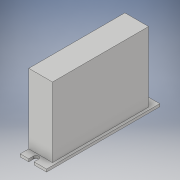
# Autodesk Inventor part: DM332T_Stepper
Saved by Autodesk Inventor 2019.4 (Build 234330000, 330)
## iProperties
Created: 2021-02-07
Part Number: DM332T_Stepper
Material: Generic
Document SubType Name: Modeling
Designer: Jorian Brusind
Density: 1 g/cm^3
Appearance: Default
Author: Jorian Brusind
Autodesk Inventor part; units mm, degrees
ref_plane "YZ Plane" through (0, 0, 0) normal (1, 0, 0) x (0, 1, 0)
ref_plane "XZ Plane" through (0, 0, 0) normal (0, 1, 0) x (-1, 0, 0)
ref_plane "XY Plane" through (0, 0, 0) normal (0, 0, 1) x (1, 0, 0)
sketch "Sketch1" plane through (0, 0, 0) normal (0, 1, 0) x (-1, 0, 0)
  line L0 (0, 0) -> (20, 0)
  line L1 (20, 0) -> (20, -86)
  line L2 (20, -86) -> (0, -86)
  line L3 (0, -86) -> (0, 0)
  dimension "d0" = 20
  dimension "d1" = 86
  constraints: 8 end point, 2 parallel, 1 horizontal, 1 perpendicular
  measures "d0" distance of L1.end L2.end
  measures "d1" distance of L0.end L1.end
extrude "Extrusion1" add sketch "Sketch1" along normal blind 2
sketch "Sketch2" plane through (0, 2, 0) normal (0, 1, 0) x (1, 0, 0)
  line L0 (0, 0) -> (0, 86) projected
  line L1 (0, 0) -> (-11.5, 0)
  line L2 (-20, 0) -> (0, 0) projected
  line L3 (-11.5, -3.5) -> (-11.5, 3.5) construction
  line L4 (-9.5, -3.5) -> (-9.5, 3.5)
  line L5 (-13.5, 3.5) -> (-13.5, -3.5)
  arc A0 (-13.5, -3.5) -> (-9.5, -3.5) centre (-11.5, -3.5) ccw
  arc A1 (-9.5, 3.5) -> (-13.5, 3.5) centre (-11.5, 3.5) ccw
  line L6 (-11.5, 89.5) -> (-11.5, 82.5) construction
  line L7 (0, 86) -> (-20, 86) projected
  line L8 (-13.5, 89.5) -> (-13.5, 82.5)
  line L9 (-9.5, 82.5) -> (-9.5, 89.5)
  arc A2 (-9.5, 89.5) -> (-13.5, 89.5) centre (-11.5, 89.5) ccw
  arc A3 (-13.5, 82.5) -> (-9.5, 82.5) centre (-11.5, 82.5) ccw
  line L10 (-11.5, 86) -> (-4.5, 86) construction
  dimension "d4" = 11.5
  dimension "d5" = 3.5
  dimension "d6" = 4
  dimension "d7" = 3.5
  dimension "d8" = 90
  dimension "d9" = 4
  dimension "d10" = 11.5
  constraints: 20 end point, 8 point on circle, 8 tangent, 4 centre point, 2 midpoint, 2 parallel, 2 perpendicular, 2 point on line, 1 horizontal, 1 vertical
  measures "d4" distance of L0.start L1.end
  measures "d5" distance of L1.end L3.end
  measures "d6" diameter of A1
  measures "d7" distance of L10.start L6.end
  measures "d8" angle of L6 L10
  measures "d9" diameter of A3
  measures "d10" distance from line of L6.end L0
extrude "Extrusion2" cut sketch "Sketch2" against normal blind 2
sketch "Sketch3" plane through (0, 2, 0) normal (0, 1, 0) x (1, 0, 0)
  arc A0 (-9.5, 3.5) -> (-13.5, 3.5) centre (-11.5, 3.5) ccw projected
  line L0 (-11.5, 3.5) -> (-11.5, 6.5)
  arc A1 (-13.5, 82.5) -> (-9.5, 82.5) centre (-11.5, 82.5) ccw projected
  line L1 (-11.5, 82.5) -> (-11.5, 79.5)
  line L2 (-11.5, 79.5) -> (-20, 79.5)
  line L3 (-20, 0) -> (-20, 86) projected
  line L4 (-11.5, 6.5) -> (-2, 6.5)
  line L5 (0, 86) -> (0, 0) projected
  line L6 (-2, 6.5) -> (-20, 6.5)
  line L7 (-20, 6.5) -> (-20, 79.5)
  line L8 (-20, 79.5) -> (-2, 79.5)
  line L9 (-2, 79.5) -> (-2, 6.5)
  dimension "d13" = 3
  dimension "d14" = 3
  dimension "d15" = 9.5
  constraints: 16 end point, 2 horizontal, 2 parallel, 2 perpendicular, 2 vertical, 1 point on line
  measures "d13" distance of L0.start L0.end
  measures "d14" distance of L1.start L1.end
  measures "d15" distance of L0.end L4.end
extrude "Extrusion3" add sketch "Sketch3" along normal blind 53
body "Solid1"
